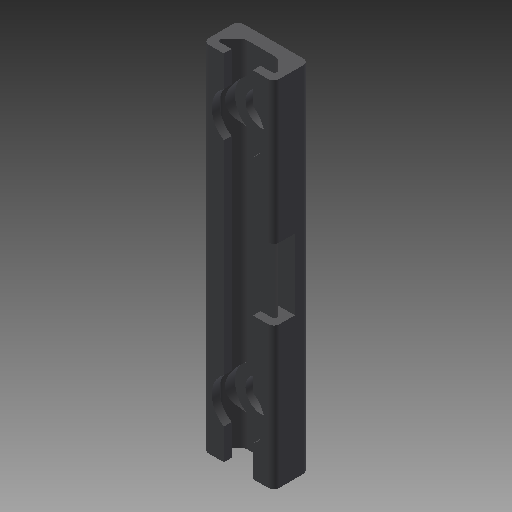
# Autodesk Inventor part: MayTec 1.68.201050_Hanging bracket
Saved by Autodesk Inventor 2018 (Build 220112000, 112)
## iProperties
Category: PARTsolutions
Company: MAYTEC
Created: 2018-01-06
Part Number: MayTec 1.68.201050_Hanging bracket
Catalog Web Link: www.cadenas.de
Description: 1.68.201050_Aufhaengung-Hanging bracket
Vendor: MAYTEC
Document SubType Name: Modeling
Designer: psAdmin
Manufacturer: MAYTEC
Mass: 10.9314 g
Surface Area: 78.5384 cm^2
Volume: 10.9314 cm^3
Density: 1 g/cm^3
Material: Generic
Appearance: PSOLRGB-175-175-175
PSOL_IDENT_0: {$CADENAS_DATA\23d-libs\maytec\maytec_3d\anbauzubehoer\aufhaengung\aufhaengung.prj},227 {VTYP=3D},{N
PSOL_IDENT_1: B=MayTec 1.68.201050_Hanging bracket},{LINA=MayTec 1.68.201050_Hanging bracket},{NN=1.68.201050_Aufh
PSOL_IDENT_2: aengung},{DATE=24.02.2017 06:59:29},{GEOMDATE=24.02.2017 06:59:25},{VERSION=},{LINEID=10},{LINESUBID=
PSOL_IDENT_3: -1},{WBVAR=}  {NB=MayTec 1.68.201050_Hanging bracket},{LINA=MayTec 1.68.201050_Hanging bracket},{KT=
PSOL_IDENT_4: DUMMY},{PARTNR=1.68.201050},{DESCRIPTION=Aufhaengung},{XTRANS=Hanging bracket}
NN: 1.68.201050_Aufhaengung
NT: Hanging bracket
NB: MayTec 1.68.201050_Hanging bracket
NBSYN: MayTec $PARTNR._$XTRANS.
LINA: MayTec 1.68.201050_Hanging bracket
PARTNR: 1.68.201050
DESCRIPTION: Hanging bracket
SUPPLIER: MAYTEC
ARTICLENO: MayTec 1.68.201050_Hanging bracket
BOMINFO: MayTec 1.68.201050_Hanging bracket
CREATOR: CADENAS GmbH
Title: MayTec 1.68.201050_Hanging bracket
Author: Cadenas PARTsolutions
Comments: Hanging bracket
Autodesk Inventor part; units mm, degrees
sketch "Skizze_1" plane through (0, 0, 0) normal (0, 1, 0) x (-1, 0, 0)
  arc A0 (10, 3.4) -> (8.4, 5) centre (8.4, 3.4) ccw
  line L0 (8.4, 5) -> (4.1, 5)
  line L1 (4.1, 5) -> (4.1, 2.8)
  line L2 (4.1, 2.8) -> (7.3, 2.8)
  arc A1 (7.795, 1.605) -> (7.3, 2.8) centre (7.3, 2.1) ccw
  line L3 (7.795, 1.605) -> (5.2757, -0.9142)
  arc A2 (3.8615, -1.5) -> (5.2757, -0.9142) centre (3.8615, 0.5) ccw
  line L4 (3.8615, -1.5) -> (-3.8615, -1.5)
  arc A3 (-5.2757, -0.9142) -> (-3.8615, -1.5) centre (-3.8615, 0.5) ccw
  line L5 (-5.2757, -0.9142) -> (-7.795, 1.605)
  arc A4 (-7.3, 2.8) -> (-7.795, 1.605) centre (-7.3, 2.1) ccw
  line L6 (-7.3, 2.8) -> (-4.1, 2.8)
  line L7 (-4.1, 2.8) -> (-4.1, 5)
  line L8 (-4.1, 5) -> (-8.4, 5)
  arc A5 (-8.4, 5) -> (-10, 3.4) centre (-8.4, 3.4) ccw
  line L9 (-10, 3.4) -> (-10, -3.4)
  arc A6 (-10, -3.4) -> (-8.4, -5) centre (-8.4, -3.4) ccw
  line L10 (-8.4, -5) -> (8.4, -5)
  arc A7 (8.4, -5) -> (10, -3.4) centre (8.4, -3.4) ccw
  line L11 (10, -3.4) -> (10, 3.4)
  constraints: 24 end point, 16 point on circle, 8 centre point
extrude "Extrusion1" add sketch "Skizze_1" along normal mid plane 100
sketch "Skizze_2" plane through (0, 0, 0) normal (1, 0, 0) x (0, 1, 0)
  line L0 (10, 9) -> (-10, 9)
  line L1 (-10, 9) -> (-10, -1)
  line L2 (-10, -1) -> (10, -1)
  line L3 (10, -1) -> (10, 9)
  constraints: 8 end point
extrude "Extrusion2" cut sketch "Skizze_2" along normal blind 15
sketch "Skizze_3_ALT_Drilling_1" plane through (0, 0, 0) normal (0, 0, 1) x (1, 0, 0)
  circle A0 centre (0, -35) radius 4.5
  constraints: 1 centre point
extrude "Extrusion3" cut sketch "Skizze_3_ALT_Drilling_1" against normal blind 10
sketch "Skizze_4_ALT_Drilling_2" plane through (0, 0, 0) normal (0, 0, 1) x (1, 0, 0)
  circle A0 centre (0, 35) radius 4.5
  constraints: 1 centre point
extrude "Extrusion4" cut sketch "Skizze_4_ALT_Drilling_2" against normal blind 10
sketch "Skizze_5_ALT_Drilling_3" plane through (0, 0, -1.5) normal (0, 0, 1) x (1, 0, 0)
  circle A0 centre (0, 35) radius 7.5
  constraints: 1 centre point
extrude "Extrusion5" cut sketch "Skizze_5_ALT_Drilling_3" along normal blind 10
sketch "Skizze_6_ALT_Drilling_4" plane through (0, 0, -1.5) normal (0, 0, 1) x (1, 0, 0)
  circle A0 centre (0, -35) radius 7.5
  constraints: 1 centre point
extrude "Extrusion6" cut sketch "Skizze_6_ALT_Drilling_4" along normal blind 10
ref_plane "side_1_XY" through (0, 0, -5) normal (0, 0, -1) x (-1, 0, 0)
ref_plane "side_1_YZ" through (0, 0, -5) normal (-1, 0, 0) x (0, 1, 0)
ref_plane "side_1_ZX" through (0, 0, -5) normal (0, 1, 0) x (0, 0, -1)
ref_plane "side_6a_XY" through (0, 35, 5) normal (0, 0, 1) x (1, 0, 0)
ref_plane "side_6a_YZ" through (0, 35, 5) normal (1, 0, 0) x (0, 1, 0)
ref_plane "side_6a_ZX" through (0, 35, 5) normal (0, 1, 0) x (0, 0, 1)
ref_plane "side_6b_XY" through (0, -35, 5) normal (0, 0, 1) x (1, 0, 0)
ref_plane "side_6b_YZ" through (0, -35, 5) normal (1, 0, 0) x (0, 1, 0)
ref_plane "side_6b_ZX" through (0, -35, 5) normal (0, 1, 0) x (0, 0, 1)
body "Solid1"
